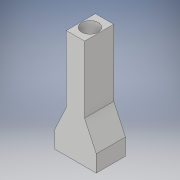
# Autodesk Inventor part: Socle P-Barre
Saved by Autodesk Inventor 2019 (Build 230136000, 136)
## iProperties
Created: 2020-03-11
Part Number: Socle P-Barre
Material: Générique
Document SubType Name: Modeling
Designer: Quentin
Density: 1 g/cm^3
Appearance: Par défaut
Author: Quentin
Autodesk Inventor part; units mm, degrees
ref_plane "YZ Plane" through (0, 0, 0) normal (1, 0, 0) x (0, 1, 0)
ref_plane "XZ Plane" through (0, 0, 0) normal (0, 1, 0) x (-1, 0, 0)
ref_plane "XY Plane" through (0, 0, 0) normal (0, 0, 1) x (1, 0, 0)
sketch "Esquisse1" plane through (0, 0, 0) normal (0, 0, 1) x (1, 0, 0)
  line L0 (0, 13) -> (-1.1, 13)
  line L1 (0, 13) -> (1.1, 13)
  line L2 (0, 0) -> (-2.5, 0)
  line L3 (0, 0) -> (2.5, 0)
  line L4 (2.5, 0) -> (2.5, 2)
  line L5 (2.5, 2) -> (1.1, 5)
  line L6 (-2.5, 0) -> (-2.5, 2)
  line L7 (-2.5, 2) -> (-1.1, 5)
  line L8 (-1.1, 5) -> (-1.1, 13)
  line L9 (1.1, 5) -> (1.1, 13)
  dimension "d0" = 13
  dimension "d1" = 1.1
  dimension "d2" = 1.1
  dimension "d3" = 8
  dimension "d5" = 2.5
  dimension "d6" = 2.5
  dimension "d7" = 2
  dimension "d8" = 2
  dimension "d18" = 8
  constraints: 20 end point, 3 horizontal, 3 vertical, 1 parallel
  measures "d0" distance of L2.start L0.start
  measures "d1" distance of L0.end L0.start
  measures "d2" distance of L1.end L0.start
  measures "d3" distance of L1.end L5.end
  measures "d5" distance of L2.start L2.end
  measures "d6" distance of L2.start L3.end
  measures "d7" distance of L3.end L4.end
  measures "d8" distance of L2.end L6.end
  measures "d18" distance of L7.end L0.end
extrude "Extrusion1" add sketch "Esquisse1" along normal blind 3.5
sketch "Esquisse3" plane through (0, 0, 0) normal (0, 0, -1) x (-1, 0, 0)
  line L0 (1.1, 5) -> (2.5, 2) projected
  line L1 (2.5, 0) -> (-2.5, 0) projected
  line L2 (2.5, 2) -> (2.5, 0) projected
  circle A0 centre (0, 1.5) radius 1.175
  line L3 (0, 0) -> (0, 1.5)
  dimension "d14" = 2.35
  dimension "d15" = 1.5
  constraints: 2 end point, 1 centre point, 1 vertical
  measures "d14" diameter of A0
  measures "d15" distance of L3.start L3.end
extrude "Extrusion3" cut sketch "Esquisse3" against normal blind 3.3
sketch "Esquisse4" plane through (-1.1, 13, 0) normal (0, 1, 0) x (1, 0, 0)
  line L0 (2.2, 0) -> (2.2, -3.5) projected
  line L1 (2.2, -1.75) -> (0, -1.75)
  line L2 (0, 0) -> (0, -3.5) projected
  circle A0 centre (1.1, -1.75) radius 1
  point P0 (1.1, 0)
  dimension "d19" = 2
  constraints: 3 midpoint, 2 end point, 1 centre point
  measures "d19" diameter of A0
extrude "Extrusion4" cut sketch "Esquisse4" against normal blind 3
